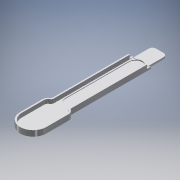
# Autodesk Inventor part: Arm
Saved by Autodesk Inventor 2016 (Build 200138000, 138)
## iProperties
Created: 2015-04-14
Part Number: Arm
Material: Generic
Document SubType Name: Modeling
Designer: Vasanth
Density: 1 g/cm^3
Appearance: Default
Mass: 21.6175 g
Surface Area: 204.007 cm^2
Volume: 21.6175 cm^3
Author: Vasanth
Autodesk Inventor part; units mm, degrees
ref_plane "YZ Plane" through (0, 0, 0) normal (1, 0, 0) x (0, 1, 0)
ref_plane "XZ Plane" through (0, 0, 0) normal (0, 1, 0) x (-1, 0, 0)
ref_plane "XY Plane" through (0, 0, 0) normal (0, 0, 1) x (1, 0, 0)
sketch "Sketch1" plane through (0, 0, 0) normal (0, 1, 0) x (-1, 0, 0)
  line L0 (52.0335, 19.2292) -> (51.733, 19.2292)
  line L1 (38.3582, 166.9806) -> (38.3582, 31.0212)
  line L2 (6.6082, 166.9806) -> (6.6082, 31.0212)
  line L3 (38.3582, 31.0212) -> (35.1832, 32.9161)
  line L4 (35.1832, 32.9161) -> (35.1832, 6.5292)
  line L5 (9.7832, 32.9161) -> (9.7832, 6.5292)
  line L6 (16.1332, 0.1792) -> (28.8332, 0.1792)
  line L7 (44.7082, 216.0792) -> (44.7082, 177.9792)
  line L8 (0.2582, 177.9792) -> (0.2582, 216.0792)
  arc A0 (44.7082, 216.0792) -> (0.2582, 216.0792) centre (22.4832, 216.0792) ccw
  arc A1 (39.9457, 169.7303) -> (38.3582, 166.9806) centre (41.5332, 166.9806) ccw
  arc A2 (28.8332, 0.1792) -> (35.1832, 6.5292) centre (28.8332, 6.5292) ccw
  arc A3 (9.7832, 6.5292) -> (16.1332, 0.1792) centre (16.1332, 6.5292) ccw
  arc A4 (39.9457, 169.7303) -> (44.7082, 177.9792) centre (35.1832, 177.9792) ccw
  arc A5 (0.2582, 177.9792) -> (5.0207, 169.7303) centre (9.7832, 177.9792) ccw
  arc A6 (6.6082, 166.9806) -> (5.0207, 169.7303) centre (3.4332, 166.9806) ccw
  line L9 (9.7832, 32.9161) -> (6.6082, 31.0212)
  dimension "d1136" = 135.9594
  dimension "d1137" = 26.3869
  dimension "d1138" = 1.8949
  dimension "d1139" = 6.35
  dimension "d1140" = 3.175
  dimension "d1141" = 9.525
  dimension "d1142" = 38.1
  dimension "d1143" = 22.225
  dimension "d1144" = 12.7
  constraints: 20 end point, 15 tangent, 14 point on circle, 7 centre point, 4 vertical, 3 equal radius, 3 parallel, 1 horizontal
  measures "d1136" distance of L2.start L2.end
  measures "d1137" distance of L5.start L5.end
  measures "d1138" vertical distance of L5.start L2.end
  measures "d1139" radius of A3
  measures "d1140" radius of A6
  measures "d1141" radius of A5
  measures "d1142" distance of L8.start L8.end
  measures "d1143" radius of A0
  measures "d1144" distance of L6.start L6.end
extrude "Extrusion1" add sketch "Sketch1" along normal blind 9.525
sketch "Sketch5" plane through (0, 9.525, 0) normal (0, 1, 0) x (1, 0, 0)
  line L0 (-52.0335, -19.2292) -> (-51.733, -19.2292)
  line L1 (-35.1832, -32.9161) -> (-35.1832, -34.2351)
  line L2 (-9.7832, -32.9161) -> (-9.7832, -34.2351)
  line L3 (-2.7995, -216.0792) -> (-2.7995, -177.9792)
  line L4 (-42.167, -216.0792) -> (-42.167, -177.9792)
  line L5 (-9.1495, -166.9806) -> (-9.1495, -34.2351)
  line L6 (-9.1495, -34.2351) -> (-9.7832, -34.2351)
  line L7 (-35.1832, -34.2351) -> (-35.9386, -34.2351)
  line L8 (-35.1832, -6.5292) -> (-35.1832, -32.9161)
  line L9 (-35.1832, -32.9161) -> (-35.1832, -6.5292) projected
  line L10 (-9.7832, -32.9161) -> (-9.7832, -6.5292)
  arc A0 (-9.7832, -6.5292) -> (-16.1332, -0.1792) centre (-16.1332, -6.5292) ccw
  arc A1 (-28.8332, -0.1792) -> (-35.1832, -6.5292) centre (-28.8332, -6.5292) ccw
  arc A2 (-38.6751, -171.9311) -> (-42.167, -177.9792) centre (-35.1832, -177.9792) ccw
  arc A3 (-2.7995, -177.9792) -> (-6.2914, -171.9311) centre (-9.7832, -177.9792) ccw
  arc A4 (-9.1495, -166.9806) -> (-6.2914, -171.9311) centre (-3.4332, -166.9806) ccw
  arc A5 (-38.6751, -171.9311) -> (-35.9386, -168.1538) centre (-41.5332, -166.9806) ccw
  line L11 (-28.8332, -0.1792) -> (-16.1332, -0.1792)
  arc A6 (-9.7832, -6.5292) -> (-16.1332, -0.1792) centre (-16.1332, -6.5292) ccw projected
  line L12 (-16.1332, -0.1792) -> (-28.8332, -0.1792) projected
  arc A7 (-42.167, -216.0792) -> (-2.7995, -216.0792) centre (-22.4832, -216.0792) ccw
  line L13 (-35.9386, -34.2351) -> (-35.9386, -168.1538)
  line L14 (-38.3582, -166.9806) -> (-38.3582, -31.0212) projected
  constraints: 24 end point, 14 point on circle, 7 centre point, 3 vertical, 2 collinear, 2 parallel, 1 horizontal, 1 point on line, 1 tangent
extrude "Extrusion2" cut sketch "Sketch5" against normal blind 6.35
sketch "Sketch6" plane through (0, 9.525, 0) normal (0, 1, 0) x (1, 0, 0)
  circle A0 centre (-22.4832, -19.2292) radius 1.5001
  circle A1 centre (-22.4832, -6.5292) radius 1.5001
  line L0 (-13.5932, -145.3906) -> (-13.5932, -112.3706)
  line L1 (-31.3732, -145.3906) -> (-31.3732, -112.3706)
  line L2 (-31.3732, -79.3506) -> (-31.3732, -46.3306)
  line L3 (-13.5932, -79.3506) -> (-13.5932, -46.3306)
  arc A2 (-13.5932, -112.3706) -> (-31.3732, -112.3706) centre (-22.4832, -112.3706) ccw
  arc A3 (-31.3732, -145.3906) -> (-13.5932, -145.3906) centre (-22.4832, -145.3906) ccw
  arc A4 (-31.3732, -79.3506) -> (-13.5932, -79.3506) centre (-22.4832, -79.3506) ccw
  arc A5 (-13.5932, -46.3306) -> (-31.3732, -46.3306) centre (-22.4832, -46.3306) ccw
  circle A6 centre (-16.8264, -221.736) radius 1.5001
  circle A7 centre (-29.2008, -222.7967) radius 1.5001
  circle A8 centre (-15.7656, -209.3616) radius 1.5001
  circle A9 centre (-22.4832, -216.0792) radius 3.5001
  circle A10 centre (-28.1401, -210.4223) radius 1.5001
  arc A11 (-15.4908, -202.4266) -> (-14.4897, -199.6071) centre (-15.4908, -200.8391) ccw
  arc A12 (-30.4768, -199.6071) -> (-29.4757, -202.4266) centre (-29.4757, -200.8391) ccw
  arc A13 (-21.4822, -193.9257) -> (-23.4843, -193.9257) centre (-22.4832, -195.1578) ccw
  arc A14 (-17.1906, -188.8121) -> (-17.1906, -191.2762) centre (-16.1895, -190.0442) ccw
  arc A15 (-7.2432, -184.0651) -> (-9.8318, -182.833) centre (-8.8307, -184.0651) ccw
  arc A16 (-9.8318, -197.2553) -> (-7.2432, -196.0232) centre (-8.8307, -196.0232) ccw
  arc A17 (-14.4897, -180.4812) -> (-15.4908, -177.6617) centre (-15.4908, -179.2492) ccw
  arc A18 (-29.4757, -177.6617) -> (-30.4768, -180.4812) centre (-29.4757, -179.2492) ccw
  arc A19 (-23.4843, -186.1626) -> (-21.4822, -186.1626) centre (-22.4832, -184.9305) ccw
  arc A20 (-27.7758, -191.2762) -> (-27.7758, -188.8121) centre (-28.7769, -190.0442) ccw
  arc A21 (-37.7232, -196.0232) -> (-35.1347, -197.2553) centre (-36.1357, -196.0232) ccw
  arc A22 (-35.1347, -182.833) -> (-37.7232, -184.0651) centre (-36.1357, -184.0651) ccw
  line L4 (-15.4908, -202.4266) -> (-29.4757, -202.4266)
  line L5 (-14.4897, -199.6071) -> (-21.4822, -193.9257)
  line L6 (-23.4843, -193.9257) -> (-30.4768, -199.6071)
  line L7 (-35.1347, -197.2553) -> (-27.7758, -191.2762)
  line L8 (-27.7758, -188.8121) -> (-35.1347, -182.833)
  line L9 (-37.7232, -184.0651) -> (-37.7232, -196.0232)
  line L10 (-30.4768, -180.4812) -> (-23.4843, -186.1626)
  line L11 (-21.4822, -186.1626) -> (-14.4897, -180.4812)
  line L12 (-15.4908, -177.6617) -> (-29.4757, -177.6617)
  line L13 (-7.2432, -196.0232) -> (-7.2432, -184.0651)
  line L14 (-9.8318, -182.833) -> (-17.1906, -188.8121)
  line L15 (-17.1906, -191.2762) -> (-9.8318, -197.2553)
  line L16 (-13.4689, -178.6236) -> (-12.1014, -178.6236) construction
  line L17 (-12.1014, -178.6236) -> (-12.1014, -180.1758) construction
  line L18 (-12.1014, -180.1758) -> (-13.4689, -180.1758) construction
  line L19 (-13.4689, -180.1758) -> (-13.4689, -178.6236) construction
  line L20 (-37.9058, -219.2042) -> (-36.1564, -219.2042) construction
  line L21 (-36.1564, -219.2042) -> (-36.1564, -220.2432) construction
  line L22 (-36.1564, -220.2432) -> (-37.9058, -220.2432) construction
  line L23 (-37.9058, -220.2432) -> (-37.9058, -219.2042) construction
  point P0 (0, 0)
  dimension "d1145" = 8.89
  dimension "d1146" = 33.02
  dimension "d1147" = 8.89
  dimension "d1148" = 3.0002
  dimension "d1149" = 3.0002
  dimension "d1150" = 8.89
  dimension "d1151" = 8.89
  dimension "d1152" = 33.02
  dimension "d1153" = 13.9849
  dimension "d1154" = 6.9925
  dimension "d1155" = 6.9925
  dimension "d1156" = 1.5875
  dimension "d1157" = 3.0002
  dimension "d1158" = 30.48
  dimension "d1159" = 24.765
  dimension "d1160" = 9.4124
  dimension "d1161" = 10.2272
  dimension "d1162" = 16
  dimension "d1163" = 11.3137
  dimension "d1164" = 7.0002
  constraints: 42 tangent, 32 end point, 32 point on circle, 23 centre point, 5 equal radius, 2 parallel, 4 other
  measures "d1145" radius of A3
  measures "d1146" distance of L0.start L0.end
  measures "d1147" radius of A2
  measures "d1148" diameter of A0
  measures "d1149" diameter of A1
  measures "d1150" radius of A5
  measures "d1151" radius of A4
  measures "d1152" distance of L3.start L3.end
  measures "d1153" distance of L12.start L12.end
  measures "d1154" horizontal distance of L10.start L10.end
  measures "d1155" horizontal distance of L11.start L11.end
  measures "d1156" radius of A18
  measures "d1157" diameter of A7
  measures "d1158" distance between parallel lines of L13 L9
  measures "d1159" distance between parallel lines of L12 L4
  measures "d1161" distance of A13.centre A19.centre
  measures "d1163" horizontal distance of A10.centre A6.centre
  measures "d1164" diameter of A9
extrude "Extrusion3" [suppressed]
sketch "Sketch7" plane through (0, 9.525, 0) normal (0, 1, 0) x (1, 0, 0)
  line L0 (-52.0335, -19.2292) -> (-51.733, -19.2292)
  line L1 (0, -16.7662) -> (-44.6659, -16.7662)
  line L2 (0, -38.112) -> (-44.6659, -38.112)
  line L3 (0, -38.112) -> (0, -16.7662)
  line L4 (-44.6659, -16.7662) -> (-44.6659, -38.112)
  point P0 (0, 0)
  constraints: 10 end point
extrude "Extrusion4" cut sketch "Sketch7" against normal blind 6.35
sketch "Sketch9" plane through (0, 9.525, 0) normal (0, 1, 0) x (1, 0, 0)
  arc A0 (-6.6082, -166.9806) -> (-5.0207, -169.7303) centre (-3.4332, -166.9806) ccw
  spline S0 degree 2 poles (-33.6688, -150.3436) (-33.6688, -161.5196) (-22.5213, -161.5196) (-11.3739, -161.5196) (-11.3739, -150.3436) knots 0 0 0 1 1 2 2 2 weights 1 0.707107 1 0.707107 1
  line L0 (-33.6688, -150.3436) -> (-33.6688, -161.5196) construction
  line L1 (-33.6688, -161.5196) -> (-22.5213, -161.5196) construction
  line L2 (-22.5213, -161.5196) -> (-11.3739, -161.5196) construction
  line L3 (-11.3739, -161.5196) -> (-11.3739, -150.3436) construction
  arc A1 (-11.3739, -41.3776) -> (-33.6688, -41.3776) centre (-22.5213, -41.3776) ccw
  line L4 (-11.3739, -150.3436) -> (-11.3739, -41.3776)
  line L5 (-33.6688, -41.3776) -> (-33.6688, -150.3436)
  point P0 (0, 0)
  constraints: 4 end point, 4 point on circle, 2 centre point, 1 parallel, 1 vertical, 3 other
extrude "Extrusion6" cut sketch "Sketch9" against normal blind 8.001
sketch "Sketch10" plane through (0, 3.175, 0) normal (0, 1, 0) x (1, 0, 0)
  line L0 (-52.0335, -19.2292) -> (-51.733, -19.2292)
  arc A0 (-38.6751, -171.9311) -> (-35.817, -166.9806) centre (-41.5332, -166.9806) ccw
  arc A1 (-38.6751, -171.9311) -> (-42.167, -177.9792) centre (-35.1832, -177.9792) ccw
  line L1 (-42.167, -177.9792) -> (-42.167, -216.0792)
  arc A2 (-42.167, -216.0792) -> (-2.7995, -216.0792) centre (-22.4832, -216.0792) ccw
  line L2 (-2.7995, -216.0792) -> (-2.7995, -177.9792)
  arc A3 (-2.7995, -177.9792) -> (-6.2914, -171.9311) centre (-9.7832, -177.9792) ccw
  arc A4 (-9.1495, -166.9806) -> (-6.2914, -171.9311) centre (-3.4332, -166.9806) ccw
  line L3 (-9.1495, -166.9806) -> (-9.1495, -34.2351)
  line L4 (-35.817, -34.2351) -> (-35.817, -166.9806)
  line L5 (-35.1832, -32.9161) -> (-35.817, -32.9161)
  line L6 (-9.7832, -32.9161) -> (-9.1495, -32.9161)
  line L7 (-9.1495, -34.2351) -> (-9.1495, -32.9161)
  line L8 (-35.817, -34.2351) -> (-35.817, -32.9161)
  line L9 (-35.1832, -32.9161) -> (-9.1495, -32.9161)
  point P0 (-9.1495, -166.9806)
  point P1 (-41.5332, -166.9806)
  point P2 (-3.4332, -166.9806)
  dimension "d1" = 0
  constraints: 20 end point, 10 point on circle, 6 tangent, 5 centre point, 2 equal radius, 2 perpendicular
extrude "Extrusion7" cut sketch "Sketch10" against normal blind 0.635
thread "Thread1" size "5-40 UNC" class "2B" standard "ANSI Unified Screw Threads" full length
thread "Thread2" size "5-40 UNC" class "2B" standard "ANSI Unified Screw Threads" full length
sketch "Sketch13" plane through (-6.6082, 0, 166.9806) normal (1, 0, 0) x (0, 0, -1)
  line L0 (0, 0) -> (0, 9.525) projected
  line L1 (0, 9.525) -> (12.7, 9.525)
  line L2 (128.8687, 9.525) -> (0, 9.525) projected
  line L3 (19.05, 4.7625) -> (19.05, 1.2573)
  line L4 (19.05, 4.7625) -> (19.05, 8.2677)
  circle A0 centre (19.05, 1.2573) radius 0.75
  circle A1 centre (19.05, 8.2677) radius 0.75
  line L5 (12.7, 8.2677) -> (19.05, 8.2677)
  point P0 (166.9806, 0)
  dimension "d1116" = 12.7
  dimension "d1117" = 3.5052
  dimension "d1118" = 3.5052
  dimension "d1119" = 1.5
  dimension "d1120" = 1.5
  dimension "d1131" = 6.35
  constraints: 8 end point, 2 centre point, 2 coincident, 1 horizontal, 1 point on line
  measures "d1116" distance of L0.end L1.end
  measures "d1117" distance of L3.start L3.end
  measures "d1118" distance of L3.start L4.end
  measures "d1119" diameter of A0
  measures "d1120" diameter of A1
  measures "d1131" distance of L5.start L5.end
sketch "Sketch14" plane through (-38.3582, 0, 31.0212) normal (-1, 0, 0) x (0, 0, 1)
  line L0 (0, 0) -> (0, 9.525)
  line L1 (0, 9.525) -> (12.7, 9.525)
  circle A0 centre (116.9094, 1.2573) radius 0.75
  circle A1 centre (116.9094, 8.2677) radius 0.75
  line L2 (7.0908, 9.525) -> (135.9594, 9.525) projected
  line L3 (135.9594, 9.525) -> (123.2594, 9.525)
  point P0 (-31.0212, 0)
  point P1 (166.9806, 0)
  dimension "d1121" = 12.7
  constraints: 6 end point, 2 centre point, 1 point on line
  measures "d1121" distance of L0.end L1.end
extrude "Extrusion9" cut sketch "Sketch14" against normal blind 0.0254
extrude "Extrusion10" cut sketch "Sketch13" against normal blind 0.0254
body "Solid1"
